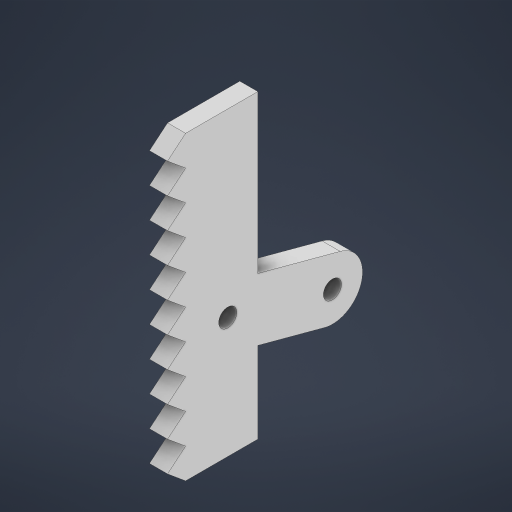
# Autodesk Inventor part: agarre_derecha
Saved by Autodesk Inventor 2023.1 (Build 271208000, 208)
## iProperties
Created: 2022-10-20
Part Number: agarre_derecha
Material: Generic
Document SubType Name: Modeling
Designer: amtat
Density: 1 g/cm^3
Appearance: Default
Author: amtat
Autodesk Inventor part; units mm, degrees
ref_plane "YZ Plane" through (0, 0, 0) normal (1, 0, 0) x (0, 1, 0)
ref_plane "XZ Plane" through (0, 0, 0) normal (0, 1, 0) x (-1, 0, 0)
ref_plane "XY Plane" through (0, 0, 0) normal (0, 0, 1) x (1, 0, 0)
sketch "Sketch1" plane through (0, 0, 0) normal (1, 0, 0) x (0, 1, 0)
  line L0 (0, 0) -> (50, 0)
  line L1 (50, 0) -> (20, 0)
  line L2 (20, 0) -> (20, 5)
  circle A0 centre (20, 5) radius 1.5
  line L3 (20, 5) -> (15.3413, -12.3867)
  line L4 (20, 5) -> (38, 5) construction
  circle A1 centre (15.3413, -12.3867) radius 1.5
  arc A2 (10.5116, -11.0926) -> (20.1709, -13.6808) centre (15.3413, -12.3867) ccw
  arc A3 (15.1704, 6.2941) -> (25, 5) centre (20, 5) ccw
  line L5 (20, 5) -> (24.8296, 3.7059)
  line L6 (15.3413, -12.3867) -> (20.1709, -13.6808)
  line L7 (20.1709, -13.6808) -> (24.8296, 3.7059)
  line L8 (20.1709, -13.6808) -> (10.5116, -11.0926)
  line L9 (24.8296, 3.7059) -> (15.1704, 6.2941)
  line L10 (15.1704, 6.2941) -> (10.5116, -11.0926)
  line L11 (0, 0) -> (0, 12)
  line L12 (0, 12) -> (50, 12)
  line L13 (50, 12) -> (50, 0)
  line L14 (50, 12) -> (45, 12)
  line L15 (45, 12) -> (40, 12)
  line L16 (40, 12) -> (35, 12)
  line L17 (35, 12) -> (30, 12)
  line L18 (30, 12) -> (25, 12)
  line L19 (25, 12) -> (20, 12)
  line L20 (20, 12) -> (15, 12)
  line L21 (15, 12) -> (10, 12)
  line L22 (10, 12) -> (5, 12)
  line L23 (5, 12) -> (0, 12)
  line L24 (50, 12) -> (47.5, 12)
  line L25 (47.5, 12) -> (47.5, 15)
  line L26 (47.5, 15) -> (50, 12)
  line L27 (47.5, 15) -> (45, 12)
  line L28 (45, 12) -> (42.5, 12)
  line L29 (42.5, 12) -> (42.5, 15)
  line L30 (42.5, 15) -> (45, 12)
  line L31 (42.5, 15) -> (40, 12)
  line L32 (40, 12) -> (37.5, 12)
  line L33 (37.5, 12) -> (37.5, 15)
  line L34 (37.5, 15) -> (40, 12)
  line L35 (37.5, 15) -> (35, 12)
  line L36 (35, 12) -> (32.5, 12)
  line L37 (32.5, 12) -> (32.5, 15)
  line L38 (32.5, 15) -> (35, 12)
  line L39 (32.5, 15) -> (30, 12)
  line L40 (30, 12) -> (27.5, 12)
  line L41 (27.5, 12) -> (27.5, 15)
  line L42 (27.5, 15) -> (30, 12)
  line L43 (27.5, 15) -> (25, 12)
  line L44 (25, 12) -> (22.5, 12)
  line L45 (22.5, 12) -> (22.5, 15)
  line L46 (22.5, 15) -> (25, 12)
  line L47 (22.5, 15) -> (20, 12)
  line L48 (20, 12) -> (17.5, 12)
  line L49 (17.5, 12) -> (17.5, 15)
  line L50 (17.5, 15) -> (20, 12)
  line L51 (17.5, 15) -> (15, 12)
  line L52 (15, 12) -> (12.5, 12)
  line L53 (12.5, 12) -> (12.5, 15)
  line L54 (12.5, 15) -> (15, 12)
  line L55 (12.5, 15) -> (10, 12)
  line L56 (10, 12) -> (7.5, 12)
  line L57 (7.5, 12) -> (7.5, 15)
  line L58 (7.5, 15) -> (10, 12)
  line L59 (7.5, 15) -> (5, 12)
  line L60 (5, 12) -> (2.5, 12)
  line L61 (2.5, 12) -> (2.5, 15)
  line L62 (2.5, 15) -> (5, 12)
  line L63 (2.5, 15) -> (0, 12)
  point P0 (23.8366, 0)
  point P1 (13.4839, 0)
  point P2 (23.8366, 0)
  dimension "d0" = 50
  dimension "d1" = 30
  dimension "d2" = 5
  dimension "d3" = 3
  dimension "d4" = 18
  dimension "d5" = 105
  dimension "d6" = 3
  dimension "d7" = 10
  dimension "d8" = 10
  dimension "d9" = 12
  dimension "d10" = 5
  dimension "d11" = 5
  dimension "d12" = 5
  dimension "d13" = 5
  dimension "d14" = 5
  dimension "d15" = 5
  dimension "d16" = 5
  dimension "d17" = 5
  dimension "d18" = 5
  dimension "d19" = 5
  dimension "d20" = 2.5
  dimension "d21" = 3
  dimension "d22" = 2.5
  dimension "d23" = 3
  dimension "d24" = 2.5
  dimension "d25" = 3
  dimension "d26" = 2.5
  dimension "d27" = 3
  dimension "d28" = 2.5
  dimension "d29" = 3
  dimension "d30" = 2.5
  dimension "d31" = 3
  dimension "d32" = 2.5
  dimension "d33" = 3
  dimension "d34" = 2.5
  dimension "d35" = 3
  dimension "d36" = 2.5
  dimension "d37" = 3
  dimension "d38" = 2.5
  dimension "d39" = 3
  constraints: 126 end point, 10 midpoint, 8 perpendicular, 7 point on line, 6 vertical, 5 point on circle, 4 centre point, 4 coincident, 3 horizontal, 2 tangent, 1 equal length, 1 parallel, 12 other
  measures "d0" distance of L0.start L0.end
  measures "d1" distance of L0.end L1.end
  measures "d2" distance of L1.end L2.end
  measures "d3" diameter of A0
  measures "d4" distance of L3.start L3.end
  measures "d5" angle of L3 L4
  measures "d6" diameter of A1
  measures "d7" diameter of A2
  measures "d8" diameter of A3
  measures "d9" distance of L0.start L11.end
  measures "d10" distance of L13.start L14.end
  measures "d11" distance of L14.end L15.end
  measures "d12" distance of L15.end L16.end
  measures "d13" distance of L16.end L17.end
  measures "d14" distance of L17.end L18.end
  measures "d15" distance of L18.end L19.end
  measures "d16" distance of L19.end L20.end
  measures "d17" distance of L20.end L21.end
  measures "d18" distance of L21.end L22.end
  measures "d19" distance of L11.end L22.end
  measures "d20" distance of L13.start L24.end
  measures "d21" distance of L24.end L25.end
  measures "d22" distance of L14.end L28.end
  measures "d23" distance of L28.end L29.end
  measures "d24" distance of L15.end L32.end
  measures "d25" distance of L32.end L33.end
  measures "d26" distance of L16.end L36.end
  measures "d27" distance of L36.end L37.end
  measures "d28" distance of L17.end L40.end
  measures "d29" distance of L40.end L41.end
  measures "d30" distance of L18.end L44.end
  measures "d31" distance of L44.end L45.end
  measures "d32" distance of L19.end L48.end
  measures "d33" distance of L48.end L49.end
  measures "d34" distance of L20.end L52.end
  measures "d35" distance of L52.end L53.end
  measures "d36" distance of L21.end L56.end
  measures "d37" distance of L56.end L57.end
  measures "d38" distance of L22.end L60.end
  measures "d39" distance of L60.end L61.end
extrude "Extrusion1" add sketch "Sketch1" along normal blind 3 contours L11 L12 L13 L0 L7 L5 A0 L9 L10 | L10 A3 L3 L0 | L0 L3 A1 L8 L10 | L63 L61 L12 | L3 A3 L0 | L0 L7 L6 A1 L3 | L9 A0 L3 A3 | L8 A1 L6 A2 | L61 L62 L12 | A3 L7 L0 | A3 L3 A0 L2 | L2 A0 L5 A3 | L59 L57 L12 | L57 L58 L12 | L55 L53 L12 | L12 L25 L26 | L53 L54 L12 | L12 L27 L25 | L51 L49 L12 | L12 L29 L30 | L49 L50 L12 | L12 L31 L29 | L47 L45 L12 | L12 L33 L34 | L45 L46 L12 | L12 L35 L33 | L43 L41 L12 | L12 L37 L38 | L41 L42 L12 | L12 L39 L37
body "Solid1"
